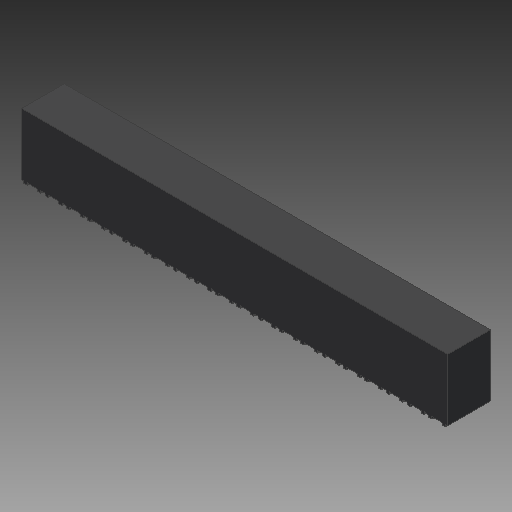
# Autodesk Inventor part: ESQ-120-33-G-D-LL_bpins
Saved by Autodesk Inventor 2019.4 (Build 234330000, 330)
## iProperties
Category: PARTsolutions
Company: SAMTEC
Created: 2017-11-11
Part Number: ESQ-120-33-G-D-LL_bpins
Catalog Web Link: www.cadenas.de
Description: ESQ Series Bottom Pins-ESQ Series - (2,54 mm) .100'' Elevated Socket
Vendor: SAMTEC
Document SubType Name: Modeling
Designer: psAdmin
Manufacturer: SAMTEC
Mass: 1.90877 g
Surface Area: 14.0387 cm^2
Volume: 1.90877 cm^3
Density: 1 g/cm^3
Material: Allgemein
Appearance: PSOLRGB-127-127-127
PSOL_IDENT_0: {$CADENAS_DATA\23d-libs\samtec\modelling\esq\parts\esq_bottom_socket.prj},214 {VTYP=3D},{NB=ESQ-120-
PSOL_IDENT_1: 33-G-D-LL_bpins},{LINA=ESQ-120-33-G-D-LL_bpins},{NN=ESQ Series Bottom Pins},{DATE=15.05.2015 12:28:0
PSOL_IDENT_2: 4},{GEOMDATE=30.12.2014 12:16:27},{VERSION=},{LINEID=10},{LINESUBID=-1},{WBVAR=POS,LS,ROW}  {NB=ESQ-
PSOL_IDENT_3: 120-33-G-D-LL_bpins},{LINA=ESQ-120-33-G-D-LL_bpins},{KT=DUMMY},{PN=ESQ-120-33-G-D-LL},{SERIES=ESQ},{
PSOL_IDENT_4: POS=20},{POSN=20},{POSALG=  '01','-01','02','-02','03','-03','04','-04','05','-05','06','-06','07','
PSOL_IDENT_5: -07','08','-08','09','-09','10','-10','11','-11','12','-12','13','-13','14','-14','15','-15','16','-
PSOL_IDENT_6: 16','17','-17','18','-18','19','-19','20','-20','21','-21','22','-22','23','-23','24','-24','25','-2
PSOL_IDENT_7: 5','26','-26','27','-27','28','-28','29','-29','30','-30','31','-31','32','-32','33','-33','34','-34'
PSOL_IDENT_8: ,'35','-35','36','-36'  },{POSPN=20},{LS=33},{PLOPT=G},{PLOPTALG= 'G','-G = 20micro\" Selective Gold
PSOL_IDENT_9: in Contact Area, 3micro\" Selective Gold on Tail.','T','-T = Matte Tin on Entire Pin.','S','-S =  3
PSOL_IDENT_10: 0micro\" Selective Gold in Contact Area, Matte Tin on Tail.','H','-H = 30micro\" Selective Gold in C
PSOL_IDENT_11: ontact Area, 3micro\" Selective Gold on Tail.','F','-F = 3micro\" Selective Gold in Contact Area, Ma
PSOL_IDENT_12: tte Tin on Tail.','E','-E = 50micro\" Selective Gold in Contact Area, 3micro\" Selective Gold on Tai
PSOL_IDENT_13: l.','L','-L = 10micro\" Selective Gold in Contact Area, Matte Tin on Tail.' },{ROW=D},{ROWPN=-D},{RO
PSOL_IDENT_14: WALG= 'S','-S = Single Row','D','-D = Double Row','T','-T = Triple Row' },{ROWN=2},{LLOPT=LL},{LLOPT
PSOL_IDENT_15: ALG= '','Not Selected','LL','-LL = Locking Lead' },{LLOPTPN=-LL},{POLOPT=},{POLOPTPN=},{POLOPTMAX=48
PSOL_IDENT_16: 0},{POLOPTMAX2='001','001','002','002','003','003','004','004','005','005','006','006','007','007','
PSOL_IDENT_17: 008','008','009','009','010','010','011','011','012','012','013','013','014','014','015','015','016'
PSOL_IDENT_18: ,'016','017','017','018','018','019','019','020','020','021','021','022','022','023','023','024','02
PSOL_IDENT_19: 4','025','025','026','026','027','027','028','028','029','029','030','030','031','031','032','032','
PSOL_IDENT_20: 033','033','034','034','035','035','036','036','037','037','038','038','039','039','040','040'},{POL
PSOL_IDENT_21: OPTALG= '','Not Selected','001','001','002','002','003','003','004','004','005','005','006','006','0
PSOL_IDENT_22: 07','007','008','008','009','009','010','010','011','011','012','012','013','013','014','014','015','
PSOL_IDENT_23: 015','016','016','017','017','018','018','019','019','020','020','021','021','022','022','023','023'
PSOL_IDENT_24: ,'024','024','025','025','026','026','027','027','028','028','029','029','030','030','031','031','03
PSOL_IDENT_25: 2','032','033','033','034','034','035','035','036','036','037','037','038','038','039','039','040','
PSOL_IDENT_26: 040'},{POLARIZE='001','001','002','002','003','003','004','004','005','005','006','006','007','007','
PSOL_IDENT_27: 008','008','009','009','010','010','011','011','012','012','013','013','014','014','015','015','016'
PSOL_IDENT_28: ,'016','017','017','018','018','019','019','020','020','021','021','022','022','023','023','024','02
PSOL_IDENT_29: 4','025','025','026','026','027','027','028','028','029','029','030','030','031','031','032','032','
PSOL_IDENT_30: 033','033','034','034','035','035','036','036','037','037','038','038','039','039','040','040','041'
PSOL_IDENT_31: ,'041','042','042','043','043','044','044','045','045','046','046','047','047','048','048','049','04
PSOL_IDENT_32: 9','050','050','051','051','052','052','053','053','054','054','055','055','056','056','057','057','
PSOL_IDENT_33: 058','058','059','059','060','060','061','061','062','062','063','063','064','064','065','065','066'
PSOL_IDENT_34: ,'066','067','067','068','068','069','069','070','070','071','071','072','072','073','073','074','07
PSOL_IDENT_35: 4','075','075','076','076','077','077','078','078','079','079','080','080','081','081','082','082','
PSOL_IDENT_36: 083','083','084','084','085','085','086','086','087','087','088','088','089','089','090','090','091'
PSOL_IDENT_37: ,'091','092','092','093','093','094','094','095','095','096','096','097','097','098','098','099','09
PSOL_IDENT_38: 9','100','100','101','101','102','102','103','103','104','104','105','105','106','106','107','107','
PSOL_IDENT_39: 108','108','109','109','110','110','111','111','112','112','113','113','114','114','115','115','116'
PSOL_IDENT_40: ,'116','117','117','118','118','119','119','120','120','121','121','122','122','123','123','124','12
PSOL_IDENT_41: 4','125','125','126','126','127','127','128','128','129','129','130','130','131','131','132','132','
PSOL_IDENT_42: 133','133','134','134','135','135','136','136','137','137','138','138','139','139','140','140','141'
PSOL_IDENT_43: ,'141','142','142','143','143','144','144','145','145','146','146','147','147','148','148','149','14
PSOL_IDENT_44: 9','150','150','151','151','152','152','153','153','154','154','155','155','156','156','157','157','
PSOL_IDENT_45: 158','158','159','159','160','160','161','161','162','162','163','163','164','164','165','165','166'
PSOL_IDENT_46: ,'166','167','167','168','168','169','169','170','170','171','171','172','172','173','173','174','17
PSOL_IDENT_47: 4','175','175','176','176','177','177','178','178','179','179','180','180','181','181','182','182','
PSOL_IDENT_48: 183','183','184','184','185','185','186','186','187','187','188','188','189','189','190','190','191'
PSOL_IDENT_49: ,'191','192','192','193','193','194','194','195','195','196','196','197','197','198','198','199','19
PSOL_IDENT_50: 9','200','200','201','201','202','202','203','203','204','204','205','205','206','206','207','207','
PSOL_IDENT_51: 208','208','209','209','210','210','211','211','212','212','213','213','214','214','215','215','216'
PSOL_IDENT_52: ,'216','217','217','218','218','219','219','220','220','221','221','222','222','223','223','224','22
PSOL_IDENT_53: 4','225','225','226','226','227','227','228','228','229','229','230','230','231','231','232','232','
PSOL_IDENT_54: 233','233','234','234','235','235','236','236','237','237','238','238','239','239','240','240','241'
PSOL_IDENT_55: ,'241','242','242','243','243','244','244','245','245','246','246','247','247','248','248','249','24
PSOL_IDENT_56: 9','250','250','251','251','252','252','253','253','254','254','255','255','256','256','257','257','
PSOL_IDENT_57: 258','258','259','259','260','260','261','261','262','262','263','263','264','264','265','265','266'
PSOL_IDENT_58: ,'266','267','267','268','268','269','269','270','270','271','271','272','272','273','273','274','27
PSOL_IDENT_59: 4','275','275','276','276','277','277','278','278','279','279','280','280','281','281','282','282','
PSOL_IDENT_60: 283','283','284','284','285','285','286','286','287','287','288','288','289','289','290','290','291'
PSOL_IDENT_61: ,'291','292','292','293','293','294','294','295','295','296','296','297','297','298','298','299','29
PSOL_IDENT_62: 9','300','300'},{POLARIZEX=0.00000},{POLARIZEY=0.00000},{POLARIZEN=0},{EVEN=0},{A=0.195},{A3DB=0.335
PSOL_IDENT_63: 00},{B=0.09000},{C=0.635},{D=0.725},{E=0.000},{W=2.02000},{ONES=0}
NN: ESQ Series Bottom Pins
NT: ESQ Series - (2,54 mm) .100'' Elevated Socket
NB: ESQ-120-33-G-D-LL_bpins
NBSYN: $PN._bpins
LINA: ESQ-120-33-G-D-LL_bpins
PN: ESQ-120-33-G-D-LL
POS: -20
LS: -33
ROW: -D = Double Row
A: 0.195
A3DB: 0.33500
C: 0.635
SUPPLIER: SAMTEC
ARTICLENO: ESQ-120-33-G-D-LL_bpins
BOMINFO: ESQ-120-33-G-D-LL_bpins
CREATOR: CADENAS GmbH
Title: ESQ-120-33-G-D-LL_bpins
Author: Cadenas PARTsolutions
Comments: ESQ Series - (2,54 mm) .100'' Elevated Socket
Autodesk Inventor part; units mm, degrees
(part 1 of 2)
sketch "Sketch_1" plane through (0, 0.254, 0) normal (0, 1, 0) x (1, 0, 0)
  line L0 (0.127, 2.54) -> (0.127, -2.54)
  line L1 (0.127, -2.54) -> (50.927, -2.54)
  line L2 (50.927, -2.54) -> (50.927, 2.54)
  line L3 (50.927, 2.54) -> (0.127, 2.54)
  constraints: 8 end point
extrude "Extrusion1" add sketch "Sketch_1" along normal blind 7.366
sketch "Sketch_2" plane through (0, 0, 0) normal (0, 1, 0) x (-1, 0, 0)
  line L0 (-0.3937, 2.032) -> (-0.3937, 2.54)
  line L1 (-0.3937, 2.54) -> (-0.7747, 2.54)
  line L2 (-0.7747, 2.54) -> (-0.7747, 2.032)
  line L3 (-0.7747, 2.032) -> (-0.3937, 2.032)
  constraints: 8 end point
extrude "Extrusion2" add sketch "Sketch_2" along normal blind 0.254
sketch "Pattern_1_SKETCH_1" plane through (1.6256, 0, 0) normal (0, 1, 0) x (1, 0, 0)
  line L0 (0.3937, -2.032) -> (0.3937, -2.54)
  line L1 (0.3937, -2.54) -> (0.7747, -2.54)
  line L2 (0.7747, -2.54) -> (0.7747, -2.032)
  line L3 (0.7747, -2.032) -> (0.3937, -2.032)
  constraints: 8 end point
sketch "Pattern_1_SKETCH_2" plane through (2.54, 0, 0) normal (0, 1, 0) x (1, 0, 0)
  line L0 (0.3937, -2.032) -> (0.3937, -2.54)
  line L1 (0.3937, -2.54) -> (0.7747, -2.54)
  line L2 (0.7747, -2.54) -> (0.7747, -2.032)
  line L3 (0.7747, -2.032) -> (0.3937, -2.032)
  constraints: 8 end point
sketch "Pattern_1_SKETCH_3" plane through (4.1656, 0, 0) normal (0, 1, 0) x (1, 0, 0)
  line L0 (0.3937, -2.032) -> (0.3937, -2.54)
  line L1 (0.3937, -2.54) -> (0.7747, -2.54)
  line L2 (0.7747, -2.54) -> (0.7747, -2.032)
  line L3 (0.7747, -2.032) -> (0.3937, -2.032)
  constraints: 8 end point
sketch "Pattern_1_SKETCH_4" plane through (5.08, 0, 0) normal (0, 1, 0) x (1, 0, 0)
  line L0 (0.3937, -2.032) -> (0.3937, -2.54)
  line L1 (0.3937, -2.54) -> (0.7747, -2.54)
  line L2 (0.7747, -2.54) -> (0.7747, -2.032)
  line L3 (0.7747, -2.032) -> (0.3937, -2.032)
  constraints: 8 end point
sketch "Pattern_1_SKETCH_5" plane through (6.7056, 0, 0) normal (0, 1, 0) x (1, 0, 0)
  line L0 (0.3937, -2.032) -> (0.3937, -2.54)
  line L1 (0.3937, -2.54) -> (0.7747, -2.54)
  line L2 (0.7747, -2.54) -> (0.7747, -2.032)
  line L3 (0.7747, -2.032) -> (0.3937, -2.032)
  constraints: 8 end point
sketch "Pattern_1_SKETCH_6" plane through (7.62, 0, 0) normal (0, 1, 0) x (1, 0, 0)
  line L0 (0.3937, -2.032) -> (0.3937, -2.54)
  line L1 (0.3937, -2.54) -> (0.7747, -2.54)
  line L2 (0.7747, -2.54) -> (0.7747, -2.032)
  line L3 (0.7747, -2.032) -> (0.3937, -2.032)
  constraints: 8 end point
sketch "Pattern_1_SKETCH_7" plane through (9.2456, 0, 0) normal (0, 1, 0) x (1, 0, 0)
  line L0 (0.3937, -2.032) -> (0.3937, -2.54)
  line L1 (0.3937, -2.54) -> (0.7747, -2.54)
  line L2 (0.7747, -2.54) -> (0.7747, -2.032)
  line L3 (0.7747, -2.032) -> (0.3937, -2.032)
  constraints: 8 end point
sketch "Pattern_1_SKETCH_8" plane through (10.16, 0, 0) normal (0, 1, 0) x (1, 0, 0)
  line L0 (0.3937, -2.032) -> (0.3937, -2.54)
  line L1 (0.3937, -2.54) -> (0.7747, -2.54)
  line L2 (0.7747, -2.54) -> (0.7747, -2.032)
  line L3 (0.7747, -2.032) -> (0.3937, -2.032)
  constraints: 8 end point
sketch "Pattern_1_SKETCH_9" plane through (11.7856, 0, 0) normal (0, 1, 0) x (1, 0, 0)
  line L0 (0.3937, -2.032) -> (0.3937, -2.54)
  line L1 (0.3937, -2.54) -> (0.7747, -2.54)
  line L2 (0.7747, -2.54) -> (0.7747, -2.032)
  line L3 (0.7747, -2.032) -> (0.3937, -2.032)
  constraints: 8 end point
sketch "Pattern_1_SKETCH_10" plane through (12.7, 0, 0) normal (0, 1, 0) x (1, 0, 0)
  line L0 (0.3937, -2.032) -> (0.3937, -2.54)
  line L1 (0.3937, -2.54) -> (0.7747, -2.54)
  line L2 (0.7747, -2.54) -> (0.7747, -2.032)
  line L3 (0.7747, -2.032) -> (0.3937, -2.032)
  constraints: 8 end point
sketch "Pattern_1_SKETCH_11" plane through (14.3256, 0, 0) normal (0, 1, 0) x (1, 0, 0)
  line L0 (0.3937, -2.032) -> (0.3937, -2.54)
  line L1 (0.3937, -2.54) -> (0.7747, -2.54)
  line L2 (0.7747, -2.54) -> (0.7747, -2.032)
  line L3 (0.7747, -2.032) -> (0.3937, -2.032)
  constraints: 8 end point
sketch "Pattern_1_SKETCH_12" plane through (15.24, 0, 0) normal (0, 1, 0) x (1, 0, 0)
  line L0 (0.3937, -2.032) -> (0.3937, -2.54)
  line L1 (0.3937, -2.54) -> (0.7747, -2.54)
  line L2 (0.7747, -2.54) -> (0.7747, -2.032)
  line L3 (0.7747, -2.032) -> (0.3937, -2.032)
  constraints: 8 end point
sketch "Pattern_1_SKETCH_13" plane through (16.8656, 0, 0) normal (0, 1, 0) x (1, 0, 0)
  line L0 (0.3937, -2.032) -> (0.3937, -2.54)
  line L1 (0.3937, -2.54) -> (0.7747, -2.54)
  line L2 (0.7747, -2.54) -> (0.7747, -2.032)
  line L3 (0.7747, -2.032) -> (0.3937, -2.032)
  constraints: 8 end point
sketch "Pattern_1_SKETCH_14" plane through (17.78, 0, 0) normal (0, 1, 0) x (1, 0, 0)
  line L0 (0.3937, -2.032) -> (0.3937, -2.54)
  line L1 (0.3937, -2.54) -> (0.7747, -2.54)
  line L2 (0.7747, -2.54) -> (0.7747, -2.032)
  line L3 (0.7747, -2.032) -> (0.3937, -2.032)
  constraints: 8 end point
sketch "Pattern_1_SKETCH_15" plane through (19.4056, 0, 0) normal (0, 1, 0) x (1, 0, 0)
  line L0 (0.3937, -2.032) -> (0.3937, -2.54)
  line L1 (0.3937, -2.54) -> (0.7747, -2.54)
  line L2 (0.7747, -2.54) -> (0.7747, -2.032)
  line L3 (0.7747, -2.032) -> (0.3937, -2.032)
  constraints: 8 end point
sketch "Pattern_1_SKETCH_16" plane through (20.32, 0, 0) normal (0, 1, 0) x (1, 0, 0)
  line L0 (0.3937, -2.032) -> (0.3937, -2.54)
  line L1 (0.3937, -2.54) -> (0.7747, -2.54)
  line L2 (0.7747, -2.54) -> (0.7747, -2.032)
  line L3 (0.7747, -2.032) -> (0.3937, -2.032)
  constraints: 8 end point
sketch "Pattern_1_SKETCH_17" plane through (21.9456, 0, 0) normal (0, 1, 0) x (1, 0, 0)
  line L0 (0.3937, -2.032) -> (0.3937, -2.54)
  line L1 (0.3937, -2.54) -> (0.7747, -2.54)
  line L2 (0.7747, -2.54) -> (0.7747, -2.032)
  line L3 (0.7747, -2.032) -> (0.3937, -2.032)
  constraints: 8 end point
sketch "Pattern_1_SKETCH_18" plane through (22.86, 0, 0) normal (0, 1, 0) x (1, 0, 0)
  line L0 (0.3937, -2.032) -> (0.3937, -2.54)
  line L1 (0.3937, -2.54) -> (0.7747, -2.54)
  line L2 (0.7747, -2.54) -> (0.7747, -2.032)
  line L3 (0.7747, -2.032) -> (0.3937, -2.032)
  constraints: 8 end point
sketch "Pattern_1_SKETCH_19" plane through (24.4856, 0, 0) normal (0, 1, 0) x (1, 0, 0)
  line L0 (0.3937, -2.032) -> (0.3937, -2.54)
  line L1 (0.3937, -2.54) -> (0.7747, -2.54)
  line L2 (0.7747, -2.54) -> (0.7747, -2.032)
  line L3 (0.7747, -2.032) -> (0.3937, -2.032)
  constraints: 8 end point
sketch "Pattern_1_SKETCH_20" plane through (25.4, 0, 0) normal (0, 1, 0) x (1, 0, 0)
  line L0 (0.3937, -2.032) -> (0.3937, -2.54)
  line L1 (0.3937, -2.54) -> (0.7747, -2.54)
  line L2 (0.7747, -2.54) -> (0.7747, -2.032)
  line L3 (0.7747, -2.032) -> (0.3937, -2.032)
  constraints: 8 end point
sketch "Pattern_1_SKETCH_21" plane through (27.0256, 0, 0) normal (0, 1, 0) x (1, 0, 0)
  line L0 (0.3937, -2.032) -> (0.3937, -2.54)
  line L1 (0.3937, -2.54) -> (0.7747, -2.54)
  line L2 (0.7747, -2.54) -> (0.7747, -2.032)
  line L3 (0.7747, -2.032) -> (0.3937, -2.032)
  constraints: 8 end point
sketch "Pattern_1_SKETCH_22" plane through (27.94, 0, 0) normal (0, 1, 0) x (1, 0, 0)
  line L0 (0.3937, -2.032) -> (0.3937, -2.54)
  line L1 (0.3937, -2.54) -> (0.7747, -2.54)
  line L2 (0.7747, -2.54) -> (0.7747, -2.032)
  line L3 (0.7747, -2.032) -> (0.3937, -2.032)
  constraints: 8 end point
sketch "Pattern_1_SKETCH_23" plane through (29.5656, 0, 0) normal (0, 1, 0) x (1, 0, 0)
  line L0 (0.3937, -2.032) -> (0.3937, -2.54)
  line L1 (0.3937, -2.54) -> (0.7747, -2.54)
  line L2 (0.7747, -2.54) -> (0.7747, -2.032)
  line L3 (0.7747, -2.032) -> (0.3937, -2.032)
  constraints: 8 end point
sketch "Pattern_1_SKETCH_24" plane through (30.48, 0, 0) normal (0, 1, 0) x (1, 0, 0)
  line L0 (0.3937, -2.032) -> (0.3937, -2.54)
  line L1 (0.3937, -2.54) -> (0.7747, -2.54)
  line L2 (0.7747, -2.54) -> (0.7747, -2.032)
  line L3 (0.7747, -2.032) -> (0.3937, -2.032)
  constraints: 8 end point
sketch "Pattern_1_SKETCH_25" plane through (32.1056, 0, 0) normal (0, 1, 0) x (1, 0, 0)
  line L0 (0.3937, -2.032) -> (0.3937, -2.54)
  line L1 (0.3937, -2.54) -> (0.7747, -2.54)
  line L2 (0.7747, -2.54) -> (0.7747, -2.032)
  line L3 (0.7747, -2.032) -> (0.3937, -2.032)
  constraints: 8 end point
sketch "Pattern_1_SKETCH_26" plane through (33.02, 0, 0) normal (0, 1, 0) x (1, 0, 0)
  line L0 (0.3937, -2.032) -> (0.3937, -2.54)
  line L1 (0.3937, -2.54) -> (0.7747, -2.54)
  line L2 (0.7747, -2.54) -> (0.7747, -2.032)
  line L3 (0.7747, -2.032) -> (0.3937, -2.032)
  constraints: 8 end point
sketch "Pattern_1_SKETCH_27" plane through (34.6456, 0, 0) normal (0, 1, 0) x (1, 0, 0)
  line L0 (0.3937, -2.032) -> (0.3937, -2.54)
  line L1 (0.3937, -2.54) -> (0.7747, -2.54)
  line L2 (0.7747, -2.54) -> (0.7747, -2.032)
  line L3 (0.7747, -2.032) -> (0.3937, -2.032)
  constraints: 8 end point
sketch "Pattern_1_SKETCH_28" plane through (35.56, 0, 0) normal (0, 1, 0) x (1, 0, 0)
  line L0 (0.3937, -2.032) -> (0.3937, -2.54)
  line L1 (0.3937, -2.54) -> (0.7747, -2.54)
  line L2 (0.7747, -2.54) -> (0.7747, -2.032)
  line L3 (0.7747, -2.032) -> (0.3937, -2.032)
  constraints: 8 end point
sketch "Pattern_1_SKETCH_29" plane through (37.1856, 0, 0) normal (0, 1, 0) x (1, 0, 0)
  line L0 (0.3937, -2.032) -> (0.3937, -2.54)
  line L1 (0.3937, -2.54) -> (0.7747, -2.54)
  line L2 (0.7747, -2.54) -> (0.7747, -2.032)
  line L3 (0.7747, -2.032) -> (0.3937, -2.032)
  constraints: 8 end point
sketch "Pattern_1_SKETCH_30" plane through (38.1, 0, 0) normal (0, 1, 0) x (1, 0, 0)
  line L0 (0.3937, -2.032) -> (0.3937, -2.54)
  line L1 (0.3937, -2.54) -> (0.7747, -2.54)
  line L2 (0.7747, -2.54) -> (0.7747, -2.032)
  line L3 (0.7747, -2.032) -> (0.3937, -2.032)
  constraints: 8 end point
sketch "Pattern_1_SKETCH_31" plane through (39.7256, 0, 0) normal (0, 1, 0) x (1, 0, 0)
  line L0 (0.3937, -2.032) -> (0.3937, -2.54)
  line L1 (0.3937, -2.54) -> (0.7747, -2.54)
  line L2 (0.7747, -2.54) -> (0.7747, -2.032)
  line L3 (0.7747, -2.032) -> (0.3937, -2.032)
  constraints: 8 end point
sketch "Pattern_1_SKETCH_32" plane through (40.64, 0, 0) normal (0, 1, 0) x (1, 0, 0)
  line L0 (0.3937, -2.032) -> (0.3937, -2.54)
  line L1 (0.3937, -2.54) -> (0.7747, -2.54)
  line L2 (0.7747, -2.54) -> (0.7747, -2.032)
  line L3 (0.7747, -2.032) -> (0.3937, -2.032)
  constraints: 8 end point
sketch "Pattern_1_SKETCH_33" plane through (42.2656, 0, 0) normal (0, 1, 0) x (1, 0, 0)
  line L0 (0.3937, -2.032) -> (0.3937, -2.54)
  line L1 (0.3937, -2.54) -> (0.7747, -2.54)
  line L2 (0.7747, -2.54) -> (0.7747, -2.032)
  line L3 (0.7747, -2.032) -> (0.3937, -2.032)
  constraints: 8 end point
sketch "Pattern_1_SKETCH_34" plane through (43.18, 0, 0) normal (0, 1, 0) x (1, 0, 0)
  line L0 (0.3937, -2.032) -> (0.3937, -2.54)
  line L1 (0.3937, -2.54) -> (0.7747, -2.54)
  line L2 (0.7747, -2.54) -> (0.7747, -2.032)
  line L3 (0.7747, -2.032) -> (0.3937, -2.032)
  constraints: 8 end point
sketch "Pattern_1_SKETCH_35" plane through (44.8056, 0, 0) normal (0, 1, 0) x (1, 0, 0)
  line L0 (0.3937, -2.032) -> (0.3937, -2.54)
  line L1 (0.3937, -2.54) -> (0.7747, -2.54)
  line L2 (0.7747, -2.54) -> (0.7747, -2.032)
  line L3 (0.7747, -2.032) -> (0.3937, -2.032)
  constraints: 8 end point
sketch "Pattern_1_SKETCH_36" plane through (45.72, 0, 0) normal (0, 1, 0) x (1, 0, 0)
  line L0 (0.3937, -2.032) -> (0.3937, -2.54)
  line L1 (0.3937, -2.54) -> (0.7747, -2.54)
  line L2 (0.7747, -2.54) -> (0.7747, -2.032)
  line L3 (0.7747, -2.032) -> (0.3937, -2.032)
  constraints: 8 end point
sketch "Pattern_1_SKETCH_37" plane through (47.3456, 0, 0) normal (0, 1, 0) x (1, 0, 0)
  line L0 (0.3937, -2.032) -> (0.3937, -2.54)
  line L1 (0.3937, -2.54) -> (0.7747, -2.54)
  line L2 (0.7747, -2.54) -> (0.7747, -2.032)
  line L3 (0.7747, -2.032) -> (0.3937, -2.032)
  constraints: 8 end point
sketch "Pattern_1_SKETCH_38" plane through (48.26, 0, 0) normal (0, 1, 0) x (1, 0, 0)
  line L0 (0.3937, -2.032) -> (0.3937, -2.54)
  line L1 (0.3937, -2.54) -> (0.7747, -2.54)
  line L2 (0.7747, -2.54) -> (0.7747, -2.032)
  line L3 (0.7747, -2.032) -> (0.3937, -2.032)
  constraints: 8 end point
sketch "Pattern_1_SKETCH_39" plane through (49.8856, 0, 0) normal (0, 1, 0) x (1, 0, 0)
  line L0 (0.3937, -2.032) -> (0.3937, -2.54)
  line L1 (0.3937, -2.54) -> (0.7747, -2.54)
  line L2 (0.7747, -2.54) -> (0.7747, -2.032)
  line L3 (0.7747, -2.032) -> (0.3937, -2.032)
  constraints: 8 end point
sketch "Pattern_1_SKETCH_40" plane through (0, 0, -4.572) normal (0, 1, 0) x (1, 0, 0)
  line L0 (0.3937, -2.032) -> (0.3937, -2.54)
  line L1 (0.3937, -2.54) -> (0.7747, -2.54)
  line L2 (0.7747, -2.54) -> (0.7747, -2.032)
  line L3 (0.7747, -2.032) -> (0.3937, -2.032)
  constraints: 8 end point
sketch "Pattern_1_SKETCH_41" plane through (1.6256, 0, -4.572) normal (0, 1, 0) x (1, 0, 0)
  line L0 (0.3937, -2.032) -> (0.3937, -2.54)
  line L1 (0.3937, -2.54) -> (0.7747, -2.54)
  line L2 (0.7747, -2.54) -> (0.7747, -2.032)
  line L3 (0.7747, -2.032) -> (0.3937, -2.032)
  constraints: 8 end point
sketch "Pattern_1_SKETCH_42" plane through (2.54, 0, -4.572) normal (0, 1, 0) x (1, 0, 0)
  line L0 (0.3937, -2.032) -> (0.3937, -2.54)
  line L1 (0.3937, -2.54) -> (0.7747, -2.54)
  line L2 (0.7747, -2.54) -> (0.7747, -2.032)
  line L3 (0.7747, -2.032) -> (0.3937, -2.032)
  constraints: 8 end point
sketch "Pattern_1_SKETCH_43" plane through (4.1656, 0, -4.572) normal (0, 1, 0) x (1, 0, 0)
  line L0 (0.3937, -2.032) -> (0.3937, -2.54)
  line L1 (0.3937, -2.54) -> (0.7747, -2.54)
  line L2 (0.7747, -2.54) -> (0.7747, -2.032)
  line L3 (0.7747, -2.032) -> (0.3937, -2.032)
  constraints: 8 end point
sketch "Pattern_1_SKETCH_44" plane through (5.08, 0, -4.572) normal (0, 1, 0) x (1, 0, 0)
  line L0 (0.3937, -2.032) -> (0.3937, -2.54)
  line L1 (0.3937, -2.54) -> (0.7747, -2.54)
  line L2 (0.7747, -2.54) -> (0.7747, -2.032)
  line L3 (0.7747, -2.032) -> (0.3937, -2.032)
  constraints: 8 end point
sketch "Pattern_1_SKETCH_45" plane through (6.7056, 0, -4.572) normal (0, 1, 0) x (1, 0, 0)
  line L0 (0.3937, -2.032) -> (0.3937, -2.54)
  line L1 (0.3937, -2.54) -> (0.7747, -2.54)
  line L2 (0.7747, -2.54) -> (0.7747, -2.032)
  line L3 (0.7747, -2.032) -> (0.3937, -2.032)
  constraints: 8 end point
sketch "Pattern_1_SKETCH_46" plane through (7.62, 0, -4.572) normal (0, 1, 0) x (1, 0, 0)
  line L0 (0.3937, -2.032) -> (0.3937, -2.54)
  line L1 (0.3937, -2.54) -> (0.7747, -2.54)
  line L2 (0.7747, -2.54) -> (0.7747, -2.032)
  line L3 (0.7747, -2.032) -> (0.3937, -2.032)
  constraints: 8 end point
sketch "Pattern_1_SKETCH_47" plane through (9.2456, 0, -4.572) normal (0, 1, 0) x (1, 0, 0)
  line L0 (0.3937, -2.032) -> (0.3937, -2.54)
  line L1 (0.3937, -2.54) -> (0.7747, -2.54)
  line L2 (0.7747, -2.54) -> (0.7747, -2.032)
  line L3 (0.7747, -2.032) -> (0.3937, -2.032)
  constraints: 8 end point
sketch "Pattern_1_SKETCH_48" plane through (10.16, 0, -4.572) normal (0, 1, 0) x (1, 0, 0)
  line L0 (0.3937, -2.032) -> (0.3937, -2.54)
  line L1 (0.3937, -2.54) -> (0.7747, -2.54)
  line L2 (0.7747, -2.54) -> (0.7747, -2.032)
  line L3 (0.7747, -2.032) -> (0.3937, -2.032)
  constraints: 8 end point
sketch "Pattern_1_SKETCH_49" plane through (11.7856, 0, -4.572) normal (0, 1, 0) x (1, 0, 0)
  line L0 (0.3937, -2.032) -> (0.3937, -2.54)
  line L1 (0.3937, -2.54) -> (0.7747, -2.54)
  line L2 (0.7747, -2.54) -> (0.7747, -2.032)
  line L3 (0.7747, -2.032) -> (0.3937, -2.032)
  constraints: 8 end point
sketch "Pattern_1_SKETCH_50" plane through (12.7, 0, -4.572) normal (0, 1, 0) x (1, 0, 0)
  line L0 (0.3937, -2.032) -> (0.3937, -2.54)
  line L1 (0.3937, -2.54) -> (0.7747, -2.54)
  line L2 (0.7747, -2.54) -> (0.7747, -2.032)
  line L3 (0.7747, -2.032) -> (0.3937, -2.032)
  constraints: 8 end point
sketch "Pattern_1_SKETCH_51" plane through (14.3256, 0, -4.572) normal (0, 1, 0) x (1, 0, 0)
  line L0 (0.3937, -2.032) -> (0.3937, -2.54)
  line L1 (0.3937, -2.54) -> (0.7747, -2.54)
  line L2 (0.7747, -2.54) -> (0.7747, -2.032)
  line L3 (0.7747, -2.032) -> (0.3937, -2.032)
  constraints: 8 end point
sketch "Pattern_1_SKETCH_52" plane through (15.24, 0, -4.572) normal (0, 1, 0) x (1, 0, 0)
  line L0 (0.3937, -2.032) -> (0.3937, -2.54)
  line L1 (0.3937, -2.54) -> (0.7747, -2.54)
  line L2 (0.7747, -2.54) -> (0.7747, -2.032)
  line L3 (0.7747, -2.032) -> (0.3937, -2.032)
  constraints: 8 end point
sketch "Pattern_1_SKETCH_53" plane through (16.8656, 0, -4.572) normal (0, 1, 0) x (1, 0, 0)
  line L0 (0.3937, -2.032) -> (0.3937, -2.54)
  line L1 (0.3937, -2.54) -> (0.7747, -2.54)
  line L2 (0.7747, -2.54) -> (0.7747, -2.032)
  line L3 (0.7747, -2.032) -> (0.3937, -2.032)
  constraints: 8 end point
sketch "Pattern_1_SKETCH_54" plane through (17.78, 0, -4.572) normal (0, 1, 0) x (1, 0, 0)
  line L0 (0.3937, -2.032) -> (0.3937, -2.54)
  line L1 (0.3937, -2.54) -> (0.7747, -2.54)
  line L2 (0.7747, -2.54) -> (0.7747, -2.032)
  line L3 (0.7747, -2.032) -> (0.3937, -2.032)
  constraints: 8 end point
sketch "Pattern_1_SKETCH_55" plane through (19.4056, 0, -4.572) normal (0, 1, 0) x (1, 0, 0)
  line L0 (0.3937, -2.032) -> (0.3937, -2.54)
  line L1 (0.3937, -2.54) -> (0.7747, -2.54)
  line L2 (0.7747, -2.54) -> (0.7747, -2.032)
  line L3 (0.7747, -2.032) -> (0.3937, -2.032)
  constraints: 8 end point
sketch "Pattern_1_SKETCH_56" plane through (20.32, 0, -4.572) normal (0, 1, 0) x (1, 0, 0)
  line L0 (0.3937, -2.032) -> (0.3937, -2.54)
  line L1 (0.3937, -2.54) -> (0.7747, -2.54)
  line L2 (0.7747, -2.54) -> (0.7747, -2.032)
  line L3 (0.7747, -2.032) -> (0.3937, -2.032)
  constraints: 8 end point
sketch "Pattern_1_SKETCH_57" plane through (21.9456, 0, -4.572) normal (0, 1, 0) x (1, 0, 0)
  line L0 (0.3937, -2.032) -> (0.3937, -2.54)
  line L1 (0.3937, -2.54) -> (0.7747, -2.54)
  line L2 (0.7747, -2.54) -> (0.7747, -2.032)
  line L3 (0.7747, -2.032) -> (0.3937, -2.032)
  constraints: 8 end point
sketch "Pattern_1_SKETCH_58" plane through (22.86, 0, -4.572) normal (0, 1, 0) x (1, 0, 0)
  line L0 (0.3937, -2.032) -> (0.3937, -2.54)
  line L1 (0.3937, -2.54) -> (0.7747, -2.54)
  line L2 (0.7747, -2.54) -> (0.7747, -2.032)
  line L3 (0.7747, -2.032) -> (0.3937, -2.032)
  constraints: 8 end point
sketch "Pattern_1_SKETCH_59" plane through (24.4856, 0, -4.572) normal (0, 1, 0) x (1, 0, 0)
  line L0 (0.3937, -2.032) -> (0.3937, -2.54)
  line L1 (0.3937, -2.54) -> (0.7747, -2.54)
  line L2 (0.7747, -2.54) -> (0.7747, -2.032)
  line L3 (0.7747, -2.032) -> (0.3937, -2.032)
  constraints: 8 end point
sketch "Pattern_1_SKETCH_60" plane through (25.4, 0, -4.572) normal (0, 1, 0) x (1, 0, 0)
  line L0 (0.3937, -2.032) -> (0.3937, -2.54)
  line L1 (0.3937, -2.54) -> (0.7747, -2.54)
  line L2 (0.7747, -2.54) -> (0.7747, -2.032)
  line L3 (0.7747, -2.032) -> (0.3937, -2.032)
  constraints: 8 end point
sketch "Pattern_1_SKETCH_61" plane through (27.0256, 0, -4.572) normal (0, 1, 0) x (1, 0, 0)
  line L0 (0.3937, -2.032) -> (0.3937, -2.54)
  line L1 (0.3937, -2.54) -> (0.7747, -2.54)
  line L2 (0.7747, -2.54) -> (0.7747, -2.032)
  line L3 (0.7747, -2.032) -> (0.3937, -2.032)
  constraints: 8 end point
sketch "Pattern_1_SKETCH_62" plane through (27.94, 0, -4.572) normal (0, 1, 0) x (1, 0, 0)
  line L0 (0.3937, -2.032) -> (0.3937, -2.54)
  line L1 (0.3937, -2.54) -> (0.7747, -2.54)
  line L2 (0.7747, -2.54) -> (0.7747, -2.032)
  line L3 (0.7747, -2.032) -> (0.3937, -2.032)
  constraints: 8 end point
sketch "Pattern_1_SKETCH_63" plane through (29.5656, 0, -4.572) normal (0, 1, 0) x (1, 0, 0)
  line L0 (0.3937, -2.032) -> (0.3937, -2.54)
  line L1 (0.3937, -2.54) -> (0.7747, -2.54)
  line L2 (0.7747, -2.54) -> (0.7747, -2.032)
  line L3 (0.7747, -2.032) -> (0.3937, -2.032)
  constraints: 8 end point
sketch "Pattern_1_SKETCH_64" plane through (30.48, 0, -4.572) normal (0, 1, 0) x (1, 0, 0)
  line L0 (0.3937, -2.032) -> (0.3937, -2.54)
  line L1 (0.3937, -2.54) -> (0.7747, -2.54)
  line L2 (0.7747, -2.54) -> (0.7747, -2.032)
  line L3 (0.7747, -2.032) -> (0.3937, -2.032)
  constraints: 8 end point
sketch "Pattern_1_SKETCH_65" plane through (32.1056, 0, -4.572) normal (0, 1, 0) x (1, 0, 0)
  line L0 (0.3937, -2.032) -> (0.3937, -2.54)
  line L1 (0.3937, -2.54) -> (0.7747, -2.54)
  line L2 (0.7747, -2.54) -> (0.7747, -2.032)
  line L3 (0.7747, -2.032) -> (0.3937, -2.032)
  constraints: 8 end point
sketch "Pattern_1_SKETCH_66" plane through (33.02, 0, -4.572) normal (0, 1, 0) x (1, 0, 0)
  line L0 (0.3937, -2.032) -> (0.3937, -2.54)
  line L1 (0.3937, -2.54) -> (0.7747, -2.54)
  line L2 (0.7747, -2.54) -> (0.7747, -2.032)
  line L3 (0.7747, -2.032) -> (0.3937, -2.032)
  constraints: 8 end point
sketch "Pattern_1_SKETCH_67" plane through (34.6456, 0, -4.572) normal (0, 1, 0) x (1, 0, 0)
  line L0 (0.3937, -2.032) -> (0.3937, -2.54)
  line L1 (0.3937, -2.54) -> (0.7747, -2.54)
  line L2 (0.7747, -2.54) -> (0.7747, -2.032)
  line L3 (0.7747, -2.032) -> (0.3937, -2.032)
  constraints: 8 end point
sketch "Pattern_1_SKETCH_68" plane through (35.56, 0, -4.572) normal (0, 1, 0) x (1, 0, 0)
  line L0 (0.3937, -2.032) -> (0.3937, -2.54)
  line L1 (0.3937, -2.54) -> (0.7747, -2.54)
  line L2 (0.7747, -2.54) -> (0.7747, -2.032)
  line L3 (0.7747, -2.032) -> (0.3937, -2.032)
  constraints: 8 end point
sketch "Pattern_1_SKETCH_69" plane through (37.1856, 0, -4.572) normal (0, 1, 0) x (1, 0, 0)
  line L0 (0.3937, -2.032) -> (0.3937, -2.54)
  line L1 (0.3937, -2.54) -> (0.7747, -2.54)
  line L2 (0.7747, -2.54) -> (0.7747, -2.032)
  line L3 (0.7747, -2.032) -> (0.3937, -2.032)
  constraints: 8 end point
sketch "Pattern_1_SKETCH_70" plane through (38.1, 0, -4.572) normal (0, 1, 0) x (1, 0, 0)
  line L0 (0.3937, -2.032) -> (0.3937, -2.54)
  line L1 (0.3937, -2.54) -> (0.7747, -2.54)
  line L2 (0.7747, -2.54) -> (0.7747, -2.032)
  line L3 (0.7747, -2.032) -> (0.3937, -2.032)
  constraints: 8 end point
sketch "Pattern_1_SKETCH_71" plane through (39.7256, 0, -4.572) normal (0, 1, 0) x (1, 0, 0)
  line L0 (0.3937, -2.032) -> (0.3937, -2.54)
  line L1 (0.3937, -2.54) -> (0.7747, -2.54)
  line L2 (0.7747, -2.54) -> (0.7747, -2.032)
  line L3 (0.7747, -2.032) -> (0.3937, -2.032)
  constraints: 8 end point
sketch "Pattern_1_SKETCH_72" plane through (40.64, 0, -4.572) normal (0, 1, 0) x (1, 0, 0)
  line L0 (0.3937, -2.032) -> (0.3937, -2.54)
  line L1 (0.3937, -2.54) -> (0.7747, -2.54)
  line L2 (0.7747, -2.54) -> (0.7747, -2.032)
  line L3 (0.7747, -2.032) -> (0.3937, -2.032)
  constraints: 8 end point
sketch "Pattern_1_SKETCH_73" plane through (42.2656, 0, -4.572) normal (0, 1, 0) x (1, 0, 0)
  line L0 (0.3937, -2.032) -> (0.3937, -2.54)
  line L1 (0.3937, -2.54) -> (0.7747, -2.54)
  line L2 (0.7747, -2.54) -> (0.7747, -2.032)
  line L3 (0.7747, -2.032) -> (0.3937, -2.032)
  constraints: 8 end point
sketch "Pattern_1_SKETCH_74" plane through (43.18, 0, -4.572) normal (0, 1, 0) x (1, 0, 0)
  line L0 (0.3937, -2.032) -> (0.3937, -2.54)
  line L1 (0.3937, -2.54) -> (0.7747, -2.54)
  line L2 (0.7747, -2.54) -> (0.7747, -2.032)
  line L3 (0.7747, -2.032) -> (0.3937, -2.032)
  constraints: 8 end point
sketch "Pattern_1_SKETCH_75" plane through (44.8056, 0, -4.572) normal (0, 1, 0) x (1, 0, 0)
  line L0 (0.3937, -2.032) -> (0.3937, -2.54)
  line L1 (0.3937, -2.54) -> (0.7747, -2.54)
  line L2 (0.7747, -2.54) -> (0.7747, -2.032)
  line L3 (0.7747, -2.032) -> (0.3937, -2.032)
  constraints: 8 end point
sketch "Pattern_1_SKETCH_76" plane through (45.72, 0, -4.572) normal (0, 1, 0) x (1, 0, 0)
  line L0 (0.3937, -2.032) -> (0.3937, -2.54)
  line L1 (0.3937, -2.54) -> (0.7747, -2.54)
  line L2 (0.7747, -2.54) -> (0.7747, -2.032)
  line L3 (0.7747, -2.032) -> (0.3937, -2.032)
  constraints: 8 end point
sketch "Pattern_1_SKETCH_77" plane through (47.3456, 0, -4.572) normal (0, 1, 0) x (1, 0, 0)
  line L0 (0.3937, -2.032) -> (0.3937, -2.54)
  line L1 (0.3937, -2.54) -> (0.7747, -2.54)
  line L2 (0.7747, -2.54) -> (0.7747, -2.032)
  line L3 (0.7747, -2.032) -> (0.3937, -2.032)
  constraints: 8 end point
sketch "Pattern_1_SKETCH_78" plane through (48.26, 0, -4.572) normal (0, 1, 0) x (1, 0, 0)
  line L0 (0.3937, -2.032) -> (0.3937, -2.54)
  line L1 (0.3937, -2.54) -> (0.7747, -2.54)
  line L2 (0.7747, -2.54) -> (0.7747, -2.032)
  line L3 (0.7747, -2.032) -> (0.3937, -2.032)
  constraints: 8 end point
sketch "Pattern_1_SKETCH_79" plane through (49.8856, 0, -4.572) normal (0, 1, 0) x (1, 0, 0)
  line L0 (0.3937, -2.032) -> (0.3937, -2.54)
  line L1 (0.3937, -2.54) -> (0.7747, -2.54)
  line L2 (0.7747, -2.54) -> (0.7747, -2.032)
  line L3 (0.7747, -2.032) -> (0.3937, -2.032)
  constraints: 8 end point
extrude "Extrusion3" add sketch "Pattern_1_SKETCH_1" along normal blind 0.254
extrude "Extrusion4" add sketch "Pattern_1_SKETCH_2" along normal blind 0.254
extrude "Extrusion5" add sketch "Pattern_1_SKETCH_3" along normal blind 0.254
extrude "Extrusion6" add sketch "Pattern_1_SKETCH_4" along normal blind 0.254
extrude "Extrusion7" add sketch "Pattern_1_SKETCH_5" along normal blind 0.254
extrude "Extrusion8" add sketch "Pattern_1_SKETCH_6" along normal blind 0.254
extrude "Extrusion9" add sketch "Pattern_1_SKETCH_7" along normal blind 0.254
extrude "Extrusion10" add sketch "Pattern_1_SKETCH_8" along normal blind 0.254
extrude "Extrusion11" add sketch "Pattern_1_SKETCH_9" along normal blind 0.254
extrude "Extrusion12" add sketch "Pattern_1_SKETCH_10" along normal blind 0.254
extrude "Extrusion13" add sketch "Pattern_1_SKETCH_11" along normal blind 0.254
extrude "Extrusion14" add sketch "Pattern_1_SKETCH_12" along normal blind 0.254
extrude "Extrusion15" add sketch "Pattern_1_SKETCH_13" along normal blind 0.254
extrude "Extrusion16" add sketch "Pattern_1_SKETCH_14" along normal blind 0.254
extrude "Extrusion17" add sketch "Pattern_1_SKETCH_15" along normal blind 0.254
extrude "Extrusion18" add sketch "Pattern_1_SKETCH_16" along normal blind 0.254
extrude "Extrusion19" add sketch "Pattern_1_SKETCH_17" along normal blind 0.254
extrude "Extrusion20" add sketch "Pattern_1_SKETCH_18" along normal blind 0.254
extrude "Extrusion21" add sketch "Pattern_1_SKETCH_19" along normal blind 0.254
extrude "Extrusion22" add sketch "Pattern_1_SKETCH_20" along normal blind 0.254
extrude "Extrusion23" add sketch "Pattern_1_SKETCH_21" along normal blind 0.254
extrude "Extrusion24" add sketch "Pattern_1_SKETCH_22" along normal blind 0.254
extrude "Extrusion25" add sketch "Pattern_1_SKETCH_23" along normal blind 0.254
extrude "Extrusion26" add sketch "Pattern_1_SKETCH_24" along normal blind 0.254
extrude "Extrusion27" add sketch "Pattern_1_SKETCH_25" along normal blind 0.254
extrude "Extrusion28" add sketch "Pattern_1_SKETCH_26" along normal blind 0.254
extrude "Extrusion29" add sketch "Pattern_1_SKETCH_27" along normal blind 0.254
extrude "Extrusion30" add sketch "Pattern_1_SKETCH_28" along normal blind 0.254
extrude "Extrusion31" add sketch "Pattern_1_SKETCH_29" along normal blind 0.254
extrude "Extrusion32" add sketch "Pattern_1_SKETCH_30" along normal blind 0.254
extrude "Extrusion33" add sketch "Pattern_1_SKETCH_31" along normal blind 0.254
extrude "Extrusion34" add sketch "Pattern_1_SKETCH_32" along normal blind 0.254
extrude "Extrusion35" add sketch "Pattern_1_SKETCH_33" along normal blind 0.254
extrude "Extrusion36" add sketch "Pattern_1_SKETCH_34" along normal blind 0.254
extrude "Extrusion37" add sketch "Pattern_1_SKETCH_35" along normal blind 0.254
extrude "Extrusion38" add sketch "Pattern_1_SKETCH_36" along normal blind 0.254
extrude "Extrusion39" add sketch "Pattern_1_SKETCH_37" along normal blind 0.254
extrude "Extrusion40" add sketch "Pattern_1_SKETCH_38" along normal blind 0.254
extrude "Extrusion41" add sketch "Pattern_1_SKETCH_39" along normal blind 0.254
extrude "Extrusion42" add sketch "Pattern_1_SKETCH_40" along normal blind 0.254
extrude "Extrusion43" add sketch "Pattern_1_SKETCH_41" along normal blind 0.254
extrude "Extrusion44" add sketch "Pattern_1_SKETCH_42" along normal blind 0.254
extrude "Extrusion45" add sketch "Pattern_1_SKETCH_43" along normal blind 0.254
extrude "Extrusion46" add sketch "Pattern_1_SKETCH_44" along normal blind 0.254
extrude "Extrusion47" add sketch "Pattern_1_SKETCH_45" along normal blind 0.254
extrude "Extrusion48" add sketch "Pattern_1_SKETCH_46" along normal blind 0.254
extrude "Extrusion49" add sketch "Pattern_1_SKETCH_47" along normal blind 0.254
extrude "Extrusion50" add sketch "Pattern_1_SKETCH_48" along normal blind 0.254
extrude "Extrusion51" add sketch "Pattern_1_SKETCH_49" along normal blind 0.254
extrude "Extrusion52" add sketch "Pattern_1_SKETCH_50" along normal blind 0.254
extrude "Extrusion53" add sketch "Pattern_1_SKETCH_51" along normal blind 0.254
extrude "Extrusion54" add sketch "Pattern_1_SKETCH_52" along normal blind 0.254
extrude "Extrusion55" add sketch "Pattern_1_SKETCH_53" along normal blind 0.254
extrude "Extrusion56" add sketch "Pattern_1_SKETCH_54" along normal blind 0.254
extrude "Extrusion57" add sketch "Pattern_1_SKETCH_55" along normal blind 0.254
extrude "Extrusion58" add sketch "Pattern_1_SKETCH_56" along normal blind 0.254
extrude "Extrusion59" add sketch "Pattern_1_SKETCH_57" along normal blind 0.254
extrude "Extrusion60" add sketch "Pattern_1_SKETCH_58" along normal blind 0.254
extrude "Extrusion61" add sketch "Pattern_1_SKETCH_59" along normal blind 0.254
extrude "Extrusion62" add sketch "Pattern_1_SKETCH_60" along normal blind 0.254
extrude "Extrusion63" add sketch "Pattern_1_SKETCH_61" along normal blind 0.254
extrude "Extrusion64" add sketch "Pattern_1_SKETCH_62" along normal blind 0.254
extrude "Extrusion65" add sketch "Pattern_1_SKETCH_63" along normal blind 0.254
extrude "Extrusion66" add sketch "Pattern_1_SKETCH_64" along normal blind 0.254
extrude "Extrusion67" add sketch "Pattern_1_SKETCH_65" along normal blind 0.254
extrude "Extrusion68" add sketch "Pattern_1_SKETCH_66" along normal blind 0.254
extrude "Extrusion69" add sketch "Pattern_1_SKETCH_67" along normal blind 0.254
extrude "Extrusion70" add sketch "Pattern_1_SKETCH_68" along normal blind 0.254
extrude "Extrusion71" add sketch "Pattern_1_SKETCH_69" along normal blind 0.254
extrude "Extrusion72" add sketch "Pattern_1_SKETCH_70" along normal blind 0.254
extrude "Extrusion73" add sketch "Pattern_1_SKETCH_71" along normal blind 0.254
extrude "Extrusion74" add sketch "Pattern_1_SKETCH_72" along normal blind 0.254
extrude "Extrusion75" add sketch "Pattern_1_SKETCH_73" along normal blind 0.254
extrude "Extrusion76" add sketch "Pattern_1_SKETCH_74" along normal blind 0.254
extrude "Extrusion77" add sketch "Pattern_1_SKETCH_75" along normal blind 0.254
extrude "Extrusion78" add sketch "Pattern_1_SKETCH_76" along normal blind 0.254
extrude "Extrusion79" add sketch "Pattern_1_SKETCH_77" along normal blind 0.254
extrude "Extrusion80" add sketch "Pattern_1_SKETCH_78" along normal blind 0.254
extrude "Extrusion81" add sketch "Pattern_1_SKETCH_79" along normal blind 0.254
sketch "Sketch_4" plane through (0, 0, 0) normal (0, 1, 0) x (-1, 0, 0)
  line L0 (-0.381, -0.508) -> (-0.381, 0.508)
  line L1 (-0.381, 0.508) -> (-0.762, 0.508)
  line L2 (-0.762, 0.508) -> (-0.762, -0.508)
  line L3 (-0.762, -0.508) -> (-0.381, -0.508)
  constraints: 8 end point
extrude "Extrusion82" add sketch "Sketch_4" along normal blind 7.366
sketch "Pattern_2_SKETCH_1" plane through (1.6256, 0, 0) normal (0, 1, 0) x (1, 0, 0)
  line L0 (0.381, 0.508) -> (0.381, -0.508)
  line L1 (0.381, -0.508) -> (0.762, -0.508)
  line L2 (0.762, -0.508) -> (0.762, 0.508)
  line L3 (0.762, 0.508) -> (0.381, 0.508)
  constraints: 8 end point
sketch "Pattern_2_SKETCH_2" plane through (2.54, 0, 0) normal (0, 1, 0) x (1, 0, 0)
  line L0 (0.381, 0.508) -> (0.381, -0.508)
  line L1 (0.381, -0.508) -> (0.762, -0.508)
  line L2 (0.762, -0.508) -> (0.762, 0.508)
  line L3 (0.762, 0.508) -> (0.381, 0.508)
  constraints: 8 end point
sketch "Pattern_2_SKETCH_3" plane through (4.1656, 0, 0) normal (0, 1, 0) x (1, 0, 0)
  line L0 (0.381, 0.508) -> (0.381, -0.508)
  line L1 (0.381, -0.508) -> (0.762, -0.508)
  line L2 (0.762, -0.508) -> (0.762, 0.508)
  line L3 (0.762, 0.508) -> (0.381, 0.508)
  constraints: 8 end point
sketch "Pattern_2_SKETCH_4" plane through (5.08, 0, 0) normal (0, 1, 0) x (1, 0, 0)
  line L0 (0.381, 0.508) -> (0.381, -0.508)
  line L1 (0.381, -0.508) -> (0.762, -0.508)
  line L2 (0.762, -0.508) -> (0.762, 0.508)
  line L3 (0.762, 0.508) -> (0.381, 0.508)
  constraints: 8 end point
sketch "Pattern_2_SKETCH_5" plane through (6.7056, 0, 0) normal (0, 1, 0) x (1, 0, 0)
  line L0 (0.381, 0.508) -> (0.381, -0.508)
  line L1 (0.381, -0.508) -> (0.762, -0.508)
  line L2 (0.762, -0.508) -> (0.762, 0.508)
  line L3 (0.762, 0.508) -> (0.381, 0.508)
  constraints: 8 end point
sketch "Pattern_2_SKETCH_6" plane through (7.62, 0, 0) normal (0, 1, 0) x (1, 0, 0)
  line L0 (0.381, 0.508) -> (0.381, -0.508)
  line L1 (0.381, -0.508) -> (0.762, -0.508)
  line L2 (0.762, -0.508) -> (0.762, 0.508)
  line L3 (0.762, 0.508) -> (0.381, 0.508)
  constraints: 8 end point
sketch "Pattern_2_SKETCH_7" plane through (9.2456, 0, 0) normal (0, 1, 0) x (1, 0, 0)
  line L0 (0.381, 0.508) -> (0.381, -0.508)
  line L1 (0.381, -0.508) -> (0.762, -0.508)
  line L2 (0.762, -0.508) -> (0.762, 0.508)
  line L3 (0.762, 0.508) -> (0.381, 0.508)
  constraints: 8 end point
sketch "Pattern_2_SKETCH_8" plane through (10.16, 0, 0) normal (0, 1, 0) x (1, 0, 0)
  line L0 (0.381, 0.508) -> (0.381, -0.508)
  line L1 (0.381, -0.508) -> (0.762, -0.508)
  line L2 (0.762, -0.508) -> (0.762, 0.508)
  line L3 (0.762, 0.508) -> (0.381, 0.508)
  constraints: 8 end point
sketch "Pattern_2_SKETCH_9" plane through (11.7856, 0, 0) normal (0, 1, 0) x (1, 0, 0)
  line L0 (0.381, 0.508) -> (0.381, -0.508)
  line L1 (0.381, -0.508) -> (0.762, -0.508)
  line L2 (0.762, -0.508) -> (0.762, 0.508)
  line L3 (0.762, 0.508) -> (0.381, 0.508)
  constraints: 8 end point
sketch "Pattern_2_SKETCH_10" plane through (12.7, 0, 0) normal (0, 1, 0) x (1, 0, 0)
  line L0 (0.381, 0.508) -> (0.381, -0.508)
  line L1 (0.381, -0.508) -> (0.762, -0.508)
  line L2 (0.762, -0.508) -> (0.762, 0.508)
  line L3 (0.762, 0.508) -> (0.381, 0.508)
  constraints: 8 end point
sketch "Pattern_2_SKETCH_11" plane through (14.3256, 0, 0) normal (0, 1, 0) x (1, 0, 0)
  line L0 (0.381, 0.508) -> (0.381, -0.508)
  line L1 (0.381, -0.508) -> (0.762, -0.508)
  line L2 (0.762, -0.508) -> (0.762, 0.508)
  line L3 (0.762, 0.508) -> (0.381, 0.508)
  constraints: 8 end point
sketch "Pattern_2_SKETCH_12" plane through (15.24, 0, 0) normal (0, 1, 0) x (1, 0, 0)
  line L0 (0.381, 0.508) -> (0.381, -0.508)
  line L1 (0.381, -0.508) -> (0.762, -0.508)
  line L2 (0.762, -0.508) -> (0.762, 0.508)
  line L3 (0.762, 0.508) -> (0.381, 0.508)
  constraints: 8 end point
sketch "Pattern_2_SKETCH_13" plane through (16.8656, 0, 0) normal (0, 1, 0) x (1, 0, 0)
  line L0 (0.381, 0.508) -> (0.381, -0.508)
  line L1 (0.381, -0.508) -> (0.762, -0.508)
  line L2 (0.762, -0.508) -> (0.762, 0.508)
  line L3 (0.762, 0.508) -> (0.381, 0.508)
  constraints: 8 end point
sketch "Pattern_2_SKETCH_14" plane through (17.78, 0, 0) normal (0, 1, 0) x (1, 0, 0)
  line L0 (0.381, 0.508) -> (0.381, -0.508)
  line L1 (0.381, -0.508) -> (0.762, -0.508)
  line L2 (0.762, -0.508) -> (0.762, 0.508)
  line L3 (0.762, 0.508) -> (0.381, 0.508)
  constraints: 8 end point
sketch "Pattern_2_SKETCH_15" plane through (19.4056, 0, 0) normal (0, 1, 0) x (1, 0, 0)
  line L0 (0.381, 0.508) -> (0.381, -0.508)
  line L1 (0.381, -0.508) -> (0.762, -0.508)
  line L2 (0.762, -0.508) -> (0.762, 0.508)
  line L3 (0.762, 0.508) -> (0.381, 0.508)
  constraints: 8 end point
sketch "Pattern_2_SKETCH_16" plane through (20.32, 0, 0) normal (0, 1, 0) x (1, 0, 0)
  line L0 (0.381, 0.508) -> (0.381, -0.508)
  line L1 (0.381, -0.508) -> (0.762, -0.508)
  line L2 (0.762, -0.508) -> (0.762, 0.508)
  line L3 (0.762, 0.508) -> (0.381, 0.508)
  constraints: 8 end point
sketch "Pattern_2_SKETCH_17" plane through (21.9456, 0, 0) normal (0, 1, 0) x (1, 0, 0)
  line L0 (0.381, 0.508) -> (0.381, -0.508)
  line L1 (0.381, -0.508) -> (0.762, -0.508)
  line L2 (0.762, -0.508) -> (0.762, 0.508)
  line L3 (0.762, 0.508) -> (0.381, 0.508)
  constraints: 8 end point
sketch "Pattern_2_SKETCH_18" plane through (22.86, 0, 0) normal (0, 1, 0) x (1, 0, 0)
  line L0 (0.381, 0.508) -> (0.381, -0.508)
  line L1 (0.381, -0.508) -> (0.762, -0.508)
  line L2 (0.762, -0.508) -> (0.762, 0.508)
  line L3 (0.762, 0.508) -> (0.381, 0.508)
  constraints: 8 end point
sketch "Pattern_2_SKETCH_19" plane through (24.4856, 0, 0) normal (0, 1, 0) x (1, 0, 0)
  line L0 (0.381, 0.508) -> (0.381, -0.508)
  line L1 (0.381, -0.508) -> (0.762, -0.508)
  line L2 (0.762, -0.508) -> (0.762, 0.508)
  line L3 (0.762, 0.508) -> (0.381, 0.508)
  constraints: 8 end point
sketch "Pattern_2_SKETCH_20" plane through (25.4, 0, 0) normal (0, 1, 0) x (1, 0, 0)
  line L0 (0.381, 0.508) -> (0.381, -0.508)
  line L1 (0.381, -0.508) -> (0.762, -0.508)
  line L2 (0.762, -0.508) -> (0.762, 0.508)
  line L3 (0.762, 0.508) -> (0.381, 0.508)
  constraints: 8 end point
sketch "Pattern_2_SKETCH_21" plane through (27.0256, 0, 0) normal (0, 1, 0) x (1, 0, 0)
  line L0 (0.381, 0.508) -> (0.381, -0.508)
  line L1 (0.381, -0.508) -> (0.762, -0.508)
  line L2 (0.762, -0.508) -> (0.762, 0.508)
  line L3 (0.762, 0.508) -> (0.381, 0.508)
  constraints: 8 end point
sketch "Pattern_2_SKETCH_22" plane through (27.94, 0, 0) normal (0, 1, 0) x (1, 0, 0)
  line L0 (0.381, 0.508) -> (0.381, -0.508)
  line L1 (0.381, -0.508) -> (0.762, -0.508)
  line L2 (0.762, -0.508) -> (0.762, 0.508)
  line L3 (0.762, 0.508) -> (0.381, 0.508)
  constraints: 8 end point
sketch "Pattern_2_SKETCH_23" plane through (29.5656, 0, 0) normal (0, 1, 0) x (1, 0, 0)
  line L0 (0.381, 0.508) -> (0.381, -0.508)
  line L1 (0.381, -0.508) -> (0.762, -0.508)
  line L2 (0.762, -0.508) -> (0.762, 0.508)
  line L3 (0.762, 0.508) -> (0.381, 0.508)
  constraints: 8 end point
sketch "Pattern_2_SKETCH_24" plane through (30.48, 0, 0) normal (0, 1, 0) x (1, 0, 0)
  line L0 (0.381, 0.508) -> (0.381, -0.508)
  line L1 (0.381, -0.508) -> (0.762, -0.508)
  line L2 (0.762, -0.508) -> (0.762, 0.508)
  line L3 (0.762, 0.508) -> (0.381, 0.508)
  constraints: 8 end point
sketch "Pattern_2_SKETCH_25" plane through (32.1056, 0, 0) normal (0, 1, 0) x (1, 0, 0)
  line L0 (0.381, 0.508) -> (0.381, -0.508)
  line L1 (0.381, -0.508) -> (0.762, -0.508)
  line L2 (0.762, -0.508) -> (0.762, 0.508)
  line L3 (0.762, 0.508) -> (0.381, 0.508)
  constraints: 8 end point
sketch "Pattern_2_SKETCH_26" plane through (33.02, 0, 0) normal (0, 1, 0) x (1, 0, 0)
  line L0 (0.381, 0.508) -> (0.381, -0.508)
  line L1 (0.381, -0.508) -> (0.762, -0.508)
  line L2 (0.762, -0.508) -> (0.762, 0.508)
  line L3 (0.762, 0.508) -> (0.381, 0.508)
  constraints: 8 end point
sketch "Pattern_2_SKETCH_27" plane through (34.6456, 0, 0) normal (0, 1, 0) x (1, 0, 0)
  line L0 (0.381, 0.508) -> (0.381, -0.508)
  line L1 (0.381, -0.508) -> (0.762, -0.508)
  line L2 (0.762, -0.508) -> (0.762, 0.508)
  line L3 (0.762, 0.508) -> (0.381, 0.508)
  constraints: 8 end point
sketch "Pattern_2_SKETCH_28" plane through (35.56, 0, 0) normal (0, 1, 0) x (1, 0, 0)
  line L0 (0.381, 0.508) -> (0.381, -0.508)
  line L1 (0.381, -0.508) -> (0.762, -0.508)
  line L2 (0.762, -0.508) -> (0.762, 0.508)
  line L3 (0.762, 0.508) -> (0.381, 0.508)
  constraints: 8 end point
sketch "Pattern_2_SKETCH_29" plane through (37.1856, 0, 0) normal (0, 1, 0) x (1, 0, 0)
  line L0 (0.381, 0.508) -> (0.381, -0.508)
  line L1 (0.381, -0.508) -> (0.762, -0.508)
  line L2 (0.762, -0.508) -> (0.762, 0.508)
  line L3 (0.762, 0.508) -> (0.381, 0.508)
  constraints: 8 end point
sketch "Pattern_2_SKETCH_30" plane through (38.1, 0, 0) normal (0, 1, 0) x (1, 0, 0)
  line L0 (0.381, 0.508) -> (0.381, -0.508)
  line L1 (0.381, -0.508) -> (0.762, -0.508)
  line L2 (0.762, -0.508) -> (0.762, 0.508)
  line L3 (0.762, 0.508) -> (0.381, 0.508)
  constraints: 8 end point
sketch "Pattern_2_SKETCH_31" plane through (39.7256, 0, 0) normal (0, 1, 0) x (1, 0, 0)
  line L0 (0.381, 0.508) -> (0.381, -0.508)
  line L1 (0.381, -0.508) -> (0.762, -0.508)
  line L2 (0.762, -0.508) -> (0.762, 0.508)
  line L3 (0.762, 0.508) -> (0.381, 0.508)
  constraints: 8 end point
sketch "Pattern_2_SKETCH_32" plane through (40.64, 0, 0) normal (0, 1, 0) x (1, 0, 0)
  line L0 (0.381, 0.508) -> (0.381, -0.508)
  line L1 (0.381, -0.508) -> (0.762, -0.508)
  line L2 (0.762, -0.508) -> (0.762, 0.508)
  line L3 (0.762, 0.508) -> (0.381, 0.508)
  constraints: 8 end point
sketch "Pattern_2_SKETCH_33" plane through (42.2656, 0, 0) normal (0, 1, 0) x (1, 0, 0)
  line L0 (0.381, 0.508) -> (0.381, -0.508)
  line L1 (0.381, -0.508) -> (0.762, -0.508)
  line L2 (0.762, -0.508) -> (0.762, 0.508)
  line L3 (0.762, 0.508) -> (0.381, 0.508)
  constraints: 8 end point
sketch "Pattern_2_SKETCH_34" plane through (43.18, 0, 0) normal (0, 1, 0) x (1, 0, 0)
  line L0 (0.381, 0.508) -> (0.381, -0.508)
  line L1 (0.381, -0.508) -> (0.762, -0.508)
  line L2 (0.762, -0.508) -> (0.762, 0.508)
  line L3 (0.762, 0.508) -> (0.381, 0.508)
  constraints: 8 end point
sketch "Pattern_2_SKETCH_35" plane through (44.8056, 0, 0) normal (0, 1, 0) x (1, 0, 0)
  line L0 (0.381, 0.508) -> (0.381, -0.508)
  line L1 (0.381, -0.508) -> (0.762, -0.508)
  line L2 (0.762, -0.508) -> (0.762, 0.508)
  line L3 (0.762, 0.508) -> (0.381, 0.508)
  constraints: 8 end point